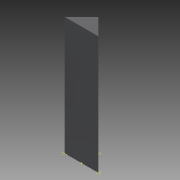
# Autodesk Inventor part: Island
Saved by Autodesk Inventor 2015 (Build 190159000, 159)
## iProperties
Created: 2015-08-24
Part Number: Island
Material: 一般
Document SubType Name: Modeling
Designer: nobuhiro
Density: 1 g/cm^3
Appearance: 滑らか - 標準の灰色
Author: nobuhiro
Autodesk Inventor part; units mm, degrees
ref_plane "YZ Plane" through (0, 0, 0) normal (1, 0, 0) x (0, 1, 0)
ref_plane "XZ Plane" through (0, 0, 0) normal (0, 1, 0) x (-1, 0, 0)
ref_plane "XY Plane" through (0, 0, 0) normal (0, 0, 1) x (1, 0, 0)
sketch "スケッチ1" plane through (0, 0, 0) normal (0, 0, 1) x (1, 0, 0)
  line L0 (-100, 0) -> (0, 100)
  line L1 (0, 100) -> (100, 0)
  line L2 (100, 0) -> (-100, 0)
  point P0 (0, 0)
  point P1 (0, 0)
  dimension "d0" = 100
  dimension "d1" = 200
  constraints: 6 end point, 2 coincident, 1 horizontal, 1 midpoint, 1 perpendicular
  measures "d0" distance from line of L2 L0.end
  measures "d1" distance of L1.end L0.start
extrude "押し出し1" add sketch "スケッチ1" along normal blind 700
sketch "スケッチ2" plane through (0, 0, 0) normal (0, 0, -1) x (-1, 0, 0)
  point P0 (0, 0)
  point P1 (0, 100)
  point P2 (100, 0)
  point P3 (-100, 0)
